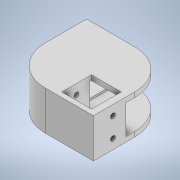
# Autodesk Inventor part: loacell_mount2
Saved by Autodesk Inventor 2022.3 (Build 263350000, 350)
## iProperties
Created: 2022-06-09
Part Number: loacell_mount2
Material: Generic
Document SubType Name: Modeling
Designer: Martijn
Density: 1 g/cm^3
Appearance: Default
Author: Martijn
Autodesk Inventor part; units mm, degrees
ref_plane "YZ Plane" through (0, 0, 0) normal (1, 0, 0) x (0, 1, 0)
ref_plane "XZ Plane" through (0, 0, 0) normal (0, 1, 0) x (-1, 0, 0)
ref_plane "XY Plane" through (0, 0, 0) normal (0, 0, 1) x (1, 0, 0)
sketch "Sketch1" plane through (0, 0, 0) normal (0, 0, 1) x (1, 0, 0)
  line L0 (0, 0) -> (44, 0)
  line L1 (44, 0) -> (44, 40)
  line L2 (44, 40) -> (0, 40)
  line L3 (0, 40) -> (0, 0)
  dimension "d0" = 44
  dimension "d1" = 40
  constraints: 8 end point, 2 parallel, 1 horizontal, 1 perpendicular
  measures "d0" distance of L0.start L0.end
  measures "d1" distance of L2.end L0.start
extrude "Extrusion1" add sketch "Sketch1" along normal blind 82
sketch "Sketch2" plane through (0, 0, 0) normal (0, -1, 0) x (1, 0, 0)
  line L0 (6.8, 77.2) -> (37.2, 77.2)
  line L1 (37.2, 77.2) -> (37.2, 46.8)
  line L2 (37.2, 46.8) -> (6.8, 46.8)
  line L3 (6.8, 46.8) -> (6.8, 77.2)
  line L4 (0, 0) -> (0, 82) projected
  line L5 (0, 82) -> (44, 82) projected
  dimension "d4" = 30.4
  dimension "d5" = 30.4
  dimension "d6" = 6.8
  dimension "d7" = 4.8
  constraints: 8 end point, 2 parallel, 1 horizontal, 1 perpendicular
  measures "d4" distance of L0.start L0.end
  measures "d5" distance of L2.end L0.start
  measures "d6" distance between parallel lines of L4 L3
  measures "d7" distance between parallel lines of L5 L0
extrude "Extrusion2" cut sketch "Sketch2" against normal blind 50
sketch "Sketch6" plane through (44, 0, 0) normal (1, 0, 0) x (0, 0, -1)
  circle A0 centre (-62.2, 30) radius 2.5
  circle A1 centre (-62.2, 10) radius 2.5
  line L0 (0, 40) -> (-82, 40) projected
  line L1 (0, 0) -> (-82, 0) projected
  point P0 (-77.2, 40)
  dimension "d24" = 5
  dimension "d25" = 10
  dimension "d26" = 5
  dimension "d27" = 10
  dimension "d28" = 15
  dimension "d29" = 15
  constraints: 2 centre point
  measures "d24" diameter of A0
  measures "d25" distance from line of L0 A0.centre
  measures "d26" diameter of A1
  measures "d27" distance from line of L1 A1.centre
  measures "d28" horizontal distance of point (-77.2, 40) A1.centre
  measures "d29" horizontal distance of point (-77.2, 40) A0.centre
extrude "Extrusion5" cut sketch "Sketch6" against normal blind 120
sketch "Sketch8" plane through (0, 0, 0) normal (-1, 0, 0) x (0, 0, 1)
  line L0 (0, 0) -> (0, 40) projected
  line L1 (77.2, 40) -> (46.8, 40) projected
  line L2 (0, 0) -> (82, 0)
  line L3 (82, 0) -> (82, 40)
  line L4 (82, 40) -> (0, 40)
  line L5 (0, 40) -> (0, 0)
  line L6 (82, 40) -> (82, 0) projected
  constraints: 8 end point, 2 parallel, 1 collinear, 1 horizontal, 1 perpendicular, 1 point on line
extrude "Extrusion7" add sketch "Sketch8" along normal blind 45
sketch "Sketch4" plane through (44, 0, 0) normal (1, 0, 0) x (0, 0, -1)
  line L0 (-6, 7.1) -> (-46.8, 7.1)
  line L1 (-46.8, 7.1) -> (-46.8, 32.9)
  line L2 (-46.8, 32.9) -> (-6, 32.9)
  line L3 (-6, 32.9) -> (-6, 7.1)
  line L4 (0, 0) -> (0, 40) projected
  line L5 (0, 0) -> (-82, 0) projected
  line L6 (-46.8, 0) -> (-46.8, 40) projected
  point P0 (0, 20)
  point P1 (-6, 20)
  dimension "d10" = 25.8
  dimension "d11" = 40.8
  dimension "d13" = 7.1
  constraints: 8 end point, 2 midpoint, 2 parallel, 1 collinear, 1 horizontal, 1 perpendicular
  measures "d10" distance between parallel lines of L0 L2
  measures "d11" distance between parallel lines of L3 L1
  measures "d13" distance between parallel lines of L5 L0
extrude "Extrusion3" cut sketch "Sketch4" against normal blind 84
sketch "Sketch5" plane through (0, 0, 0) normal (0, 0, -1) x (-1, 0, 0)
  circle A0 centre (34.2, 20) radius 3.1
  circle A1 centre (15.2, 20) radius 3.1
  line L0 (-44, 40) -> (0, 40) projected
  line L1 (45, 40) -> (45, 0) projected
  point P0 (0, 0)
  dimension "d16" = 6.2
  dimension "d17" = 6.2
  dimension "d18" = 20
  dimension "d19" = 20
  dimension "d21" = 19
  dimension "d40" = 10.8
  constraints: 2 centre point
  measures "d16" diameter of A0
  measures "d17" diameter of A1
  measures "d18" distance from line of L0 A0.centre
  measures "d19" distance from line of L0 A1.centre
  measures "d21" distance of A0.centre A1.centre
  measures "d40" distance from line of L1 A0.centre
extrude "Extrusion4" cut sketch "Sketch5" against normal blind 34
sketch "Sketch9" plane through (44, 7.1, 6) normal (0, 0, 1) x (1, 0, 0)
  line L0 (0, 25.8) -> (-84, 25.8) projected
  line L1 (0, 0) -> (-84, 0) projected
  line L2 (0, 25.8) -> (-50, 25.8)
  line L3 (-50, 25.8) -> (-50, 0)
  line L4 (-50, 0) -> (0, 0)
  line L5 (0, 0) -> (0, 25.8)
  line L6 (-84, 25.8) -> (-84, 0) projected
  point P0 (-44, -7.1)
  point P1 (-50, 25.8)
  point P2 (-84, 0)
  dimension "d41" = 34
  constraints: 8 end point, 2 parallel, 1 horizontal, 1 perpendicular, 1 point on line
  measures "d41" distance between parallel lines of L3 L6
extrude "Extrusion8" cut sketch "Sketch9" against normal blind 10 contours L5 L1 L3 L0
sketch "Sketch10" plane through (44, 0, 82) normal (1, 0, 0) x (0, 0, -1)
  line L0 (33.2, 5.1) -> (82, 5.1)
  line L1 (82, 5.1) -> (82, 34.9)
  line L2 (82, 34.9) -> (33.2, 34.9)
  line L3 (33.2, 34.9) -> (33.2, 5.1)
  line L4 (35.2, 7.1) -> (35.2, 32.9) projected
  line L5 (82, 7.1) -> (35.2, 7.1) projected
  line L6 (35.2, 32.9) -> (82, 32.9) projected
  point P0 (82, 0)
  dimension "d44" = 2
  dimension "d45" = 2
  dimension "d46" = 2
  constraints: 8 end point, 2 parallel, 1 horizontal, 1 perpendicular
  measures "d44" distance between parallel lines of L4 L3
  measures "d45" distance between parallel lines of L5 L0
  measures "d46" distance between parallel lines of L2 L6
extrude "Extrusion9" cut sketch "Sketch10" against normal up to surface (50 mm away) contours L3 L2 L1 L6 L4 L5 L0
fillet "Fillet1" radius 40 3 edges at (44, 2.55, 0) (44, 37.45, 0) (-45, 20, 82)
sketch "Sketch11" plane through (-40, 0, 0) normal (1, 0, 0) x (0, 0, -1)
  circle A0 centre (-31, 20.4) radius 3.5
  line L0 (-6, 32.9) -> (0, 32.9) projected
  line L1 (-6, 7.1) -> (-6, 32.9) projected
  line L2 (-46.8, 32.9) -> (-6, 32.9) projected
  point P0 (0, 0)
  point P1 (-46.8, 32.7)
  point P2 (-6, 20)
  point P3 (0, 32.9)
  dimension "d50" = 7
  dimension "d52" = 25
  dimension "d55" = 12.5
  constraints: 1 centre point, 1 midpoint, 2 other
  measures "d50" diameter of A0
  measures "d52" horizontal distance of point (-6, 20) A0.centre
extrude "Extrusion10" cut sketch "Sketch11" against normal blind 109
sketch "Sketch12" plane through (0, 30, 62.2) normal (1, 0, 0) x (0, 0, -1)
  circle A0 centre (0, 0) radius 6
  circle A1 centre (0, -20) radius 6
  circle A2 centre (0, -20) radius 2.5 projected
  circle A3 centre (0, 0) radius 2.5 projected
  point P0 (62.2, -30)
  dimension "d56" = 12
  dimension "d57" = 12
  constraints: 2 centre point, 2 concentric
  measures "d56" diameter of A1
  measures "d57" diameter of A0
extrude "Extrusion11" cut sketch "Sketch12" against normal blind 120 contours A0 | A1 | A2 | A3
body "Solid1"
